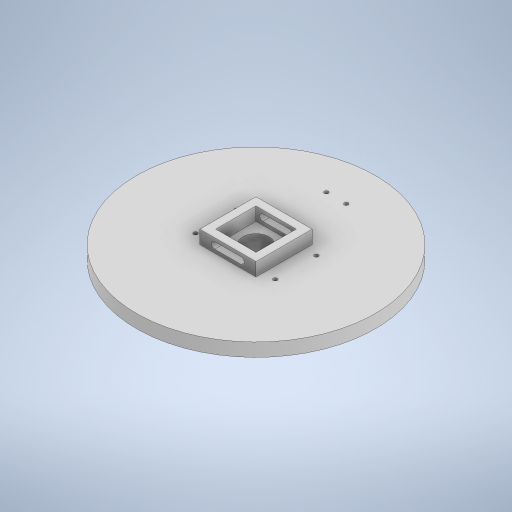
# Autodesk Inventor part: Satellite_plate
Saved by Autodesk Inventor 2023 (Build 270158000, 158)
## iProperties
Created: 2022-12-10
Part Number: Satellite_plate
Material: Generic
Document SubType Name: Modeling
Designer: Krzysztof
Density: 1 g/cm^3
Appearance: Default
Mass: 261.478 g
Surface Area: 622.91 cm^2
Volume: 261.478 cm^3
Author: Krzysztof
## iProperties of the stored document Satellite_plate_3DPrint.ipt
Created: 2022-12-19
Part Number: Satellite_plate_3DPrint
Material: Generic
Document SubType Name: Modeling
Designer: Krzysztof
Density: 1 g/cm^3
Appearance: Default
Author: Krzysztof
Autodesk Inventor part; units mm, degrees
ref_plane "YZ Plane" through (0, 0, 0) normal (1, 0, 0) x (0, 1, 0)
ref_plane "XZ Plane" through (0, 0, 0) normal (0, 1, 0) x (-1, 0, 0)
ref_plane "XY Plane" through (0, 0, 0) normal (0, 0, 1) x (1, 0, 0)
sketch "Sketch1" plane through (0, 0, 0) normal (0, 1, 0) x (-1, 0, 0)
  circle A0 centre (0, 0) radius 90
  line L0 (21.15, 21.15) -> (-21.15, 21.15) construction
  line L1 (-21.15, 21.15) -> (-21.15, -21.15) construction
  line L2 (-21.15, -21.15) -> (21.15, -21.15) construction
  line L3 (21.15, -21.15) -> (21.15, 21.15) construction
  line L4 (21.15, 21.15) -> (-21.15, -21.15) construction
  line L5 (-21.15, 21.15) -> (21.15, -21.15) construction
  circle A1 centre (0, 0) radius 10
  dimension "d0" = 180
  dimension "d1" = 42.3
  dimension "d2" = 42.3
  dimension "d3" = 20
  constraints: 12 end point, 2 centre point, 2 coincident, 2 midpoint, 2 parallel, 1 horizontal, 1 perpendicular
  measures "d0" diameter of A0
  measures "d1" distance of L1.end L2.end
  measures "d2" distance of L0.end L1.end
  measures "d3" diameter of A1
extrude "Extrusion1" add sketch "Sketch1" along normal blind 10
sketch "Sketch2" plane through (0, 0, 0) normal (0, -1, 0) x (1, 0, 0)
  circle A0 centre (0, 0) radius 15
  circle A1 centre (0, 0) radius 10
  dimension "d6" = 30
  dimension "d7" = 20
  constraints: 2 centre point, 2 coincident
  measures "d6" diameter of A0
  measures "d7" diameter of A1
extrude "Extrusion2" add sketch "Sketch2" along normal blind 3
sketch "Sketch3" plane through (0, -3, 0) normal (0, -1, 0) x (1, 0, 0)
  circle A0 centre (0, 0) radius 10
  circle A1 centre (0, 0) radius 12.5
  dimension "d10" = 25
  dimension "d11" = 20
  constraints: 2 centre point, 2 coincident
  measures "d10" diameter of A1
  measures "d11" diameter of A0
extrude "Extrusion3" add sketch "Sketch3" along normal blind 12
sketch "Sketch4" plane through (0, 10, 0) normal (0, 1, 0) x (1, 0, 0)
  line L0 (-21.15, -21.15) -> (21.15, -21.15)
  line L1 (21.15, -21.15) -> (21.15, 21.15)
  line L2 (21.15, 21.15) -> (-21.15, 21.15)
  line L3 (-21.15, 21.15) -> (-21.15, -21.15)
  line L4 (-21.15, -21.15) -> (21.15, 21.15) construction
  line L5 (21.15, -21.15) -> (-21.15, 21.15) construction
  line L6 (-15.15, -15.15) -> (15.15, -15.15)
  line L7 (15.15, -15.15) -> (15.15, 15.15)
  line L8 (15.15, 15.15) -> (-15.15, 15.15)
  line L9 (-15.15, 15.15) -> (-15.15, -15.15)
  line L10 (-15.15, -15.15) -> (15.15, 15.15) construction
  line L11 (15.15, -15.15) -> (-15.15, 15.15) construction
  point P0 (0, 0)
  dimension "d14" = 42.3
  dimension "d15" = 42.3
  dimension "d16" = 6
  constraints: 24 end point, 4 midpoint, 4 parallel, 2 horizontal, 2 perpendicular, 1 point on line
  measures "d14" distance of L1.end L2.end
  measures "d15" distance of L0.end L1.end
  measures "d16" distance between parallel lines of L2 L8
extrude "Extrusion4" add sketch "Sketch4" along normal blind 10
sketch "Sketch5" plane through (21.15, 10, -21.15) normal (0, 0, -1) x (-1, 0, 0)
  line L0 (11.15, 5) -> (31.15, 5) construction
  line L1 (11.15, 2.5) -> (31.15, 2.5)
  line L2 (31.15, 7.5) -> (11.15, 7.5)
  arc A0 (11.15, 7.5) -> (11.15, 2.5) centre (11.15, 5) ccw
  arc A1 (31.15, 2.5) -> (31.15, 7.5) centre (31.15, 5) ccw
  line L3 (0, 10) -> (42.3, 10) projected
  point P0 (21.15, -10)
  point P1 (21.15, 5)
  dimension "d19" = 5
  dimension "d20" = 20
  dimension "d21" = 2.5
  constraints: 8 end point, 4 point on circle, 4 tangent, 2 centre point, 1 horizontal, 1 midpoint, 1 parallel, 1 vertical alignment
  measures "d19" distance between parallel lines of L1 L2
  measures "d20" distance of L0.start L0.end
  measures "d21" distance between parallel lines of L3 L2
extrude "Extrusion5" cut sketch "Sketch5" against normal through all
sketch "Sketch6" plane through (0, 10, 0) normal (0, 1, 0) x (1, 0, 0)
  circle A0 centre (-30, 15.5) radius 1.5
  line L0 (0, 0) -> (41.4965, 0) construction
  line L1 (0, 0) -> (0, 38.6106) construction
  circle A1 centre (30, 15.5) radius 1.5
  circle A2 centre (-30, -15.5) radius 1.5
  circle A3 centre (30, -15.5) radius 1.5
  line L2 (-9.5, 62.5) -> (9.5, 62.5) construction
  line L3 (9.5, 62.5) -> (9.5, 47.5) construction
  line L4 (9.5, 47.5) -> (-9.5, 47.5) construction
  line L5 (-9.5, 47.5) -> (-9.5, 62.5) construction
  line L6 (-9.5, 62.5) -> (9.5, 47.5) construction
  line L7 (9.5, 62.5) -> (-9.5, 47.5) construction
  circle A4 centre (-7.5, 60.5) radius 1.5
  circle A5 centre (7.5, 60.5) radius 1.5
  point P0 (0, 55)
  dimension "d24" = 3
  dimension "d25" = 30
  dimension "d26" = 15.5
  dimension "d29" = 60
  dimension "d32" = 31
  dimension "d35" = 15
  dimension "d36" = 19
  dimension "d37" = 55
  dimension "d38" = 2
  dimension "d39" = 2
  dimension "d40" = 3
  constraints: 16 end point, 6 centre point, 3 horizontal, 2 midpoint, 2 parallel, 2 vertical, 1 perpendicular, 1 point on line, 1 symmetric about line, 7 other
  measures "d24" diameter of A0
  measures "d25" horizontal distance of A0.centre L0.start
  measures "d26" vertical distance of L0.start A0.centre
  measures "d29" distance of A0.centre A1.centre
  measures "d32" distance of A0.centre A2.centre
  measures "d35" distance of L2.end L3.end
  measures "d36" distance of L2.start L2.end
  measures "d37" distance of L0.start point (0, 55)
  measures "d38" distance from line of L2 A4.centre
  measures "d39" distance from line of L5 A4.centre
  measures "d40" diameter of A4
extrude "Extrusion6" cut sketch "Sketch6" against normal through all
equation "\"d2\" = d1"
equation "\"d15\" = d14"
body "Solid1"
